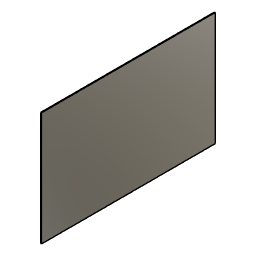
OpenBook_3D_Model (Autodesk Fusion 360 archive; units mm, degrees)
design "EPD"
Autodesk Fusion 360 part; units mm, degrees
sketch "Sketch1" plane through (0, 0, 0) normal (1, 0, 0) x (0, 1, 0)
  line L0 (0, 0) -> (170.2, 0)
  line L1 (170.2, 0) -> (170.2, 111.2)
  line L2 (170.2, 111.2) -> (0, 111.2)
  line L3 (0, 111.2) -> (0, 0)
  dimension "d1" = 170.2
  dimension "d2" = 111.2
  constraint coincident L0.start L3.end
  constraint horizontal L0
  constraint perpendicular L0 L1
  constraint perpendicular L1 L2
  constraint perpendicular L0 L3
  measures "d1" distance of L0.start L0.end
  measures "d2" distance of L0.end L1.end
extrude "Extrude1" add sketch "Sketch1" along normal blind 0.7

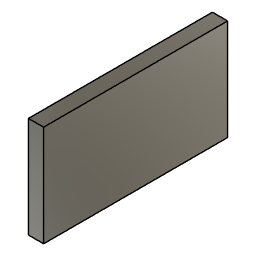
design "battery"
Autodesk Fusion 360 part; units mm, degrees
sketch "Sketch1" plane through (0, 0, 0) normal (1, 0, 0) x (0, 1, 0)
  line L0 (0, 0) -> (76.5, 0)
  line L1 (76.5, 0) -> (76.5, 42)
  line L2 (76.5, 42) -> (0, 42)
  line L3 (0, 42) -> (0, 0)
  dimension "d1" = 76.5
  dimension "d2" = 42
  constraint coincident L0.start L3.end
  constraint horizontal L0
  constraint perpendicular L0 L1
  constraint perpendicular L1 L2
  constraint perpendicular L0 L3
  measures "d1" distance of L0.start L0.end
  measures "d2" distance of L0.end L1.end
extrude "Extrude1" add sketch "Sketch1" along normal blind 6.3
